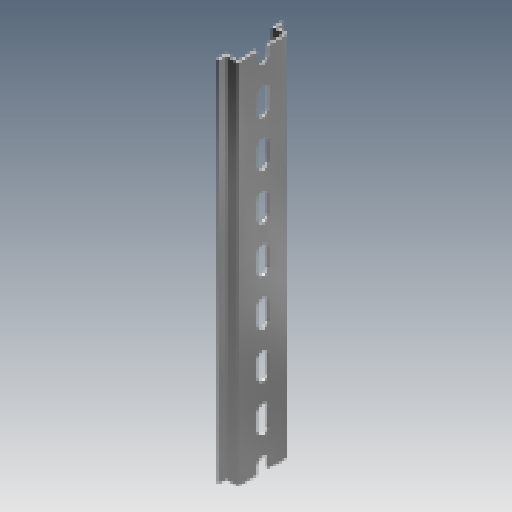
# Autodesk Inventor part: din_rail
Saved by Autodesk Inventor 2025.4 (Build 294407020, 407B)
## iProperties
Created: 2026-09-16
Part Number: din_rail
Material: Generic
Document SubType Name: Modeling
Designer: Aiden
Density: 1 g/cm^3
Appearance: Default
Author: Aiden
Autodesk Inventor part; units mm, degrees
ref_plane "YZ Plane" through (0, 0, 0) normal (1, 0, 0) x (0, 1, 0)
ref_plane "XZ Plane" through (0, 0, 0) normal (0, 1, 0) x (-1, 0, 0)
ref_plane "XY Plane" through (0, 0, 0) normal (0, 0, 1) x (1, 0, 0)
sketch "Sketch1" plane through (0, 0, 0) normal (0, 1, 0) x (-1, 0, 0)
  line L0 (0, 0) -> (0, -13.5)
  line L1 (0, -13.5) -> (6.5, -13.5)
  line L2 (6.5, -13.5) -> (6.5, -17.5)
  line L3 (1, 0) -> (1, -12.5)
  line L4 (1, -12.5) -> (7.5, -12.5)
  line L5 (7.5, -12.5) -> (7.5, -17.5)
  line L6 (7.5, -17.5) -> (6.5, -17.5)
  line L7 (1, 0) -> (0, 0) construction
  line L8 (0, 0) -> (0, 13.5)
  line L9 (0, 13.5) -> (6.5, 13.5)
  line L10 (6.5, 13.5) -> (6.5, 17.5)
  line L11 (1, 0) -> (1, 12.5)
  line L12 (1, 12.5) -> (7.5, 12.5)
  line L13 (7.5, 12.5) -> (7.5, 17.5)
  line L14 (7.5, 17.5) -> (6.5, 17.5)
  dimension "d0" = 13.5
  dimension "d1" = 1
  dimension "d2" = 7.5
  dimension "d3" = 17.5
  constraints: 30 end point, 6 symmetric about line, 3 horizontal, 2 vertical, 2 other
  measures "d0" distance of L0.start L0.end
  measures "d1" distance between parallel lines of L0 L3
  measures "d2" distance between parallel lines of L0 L5
  measures "d3" vertical distance of L2.end L0.start
extrude "Extrusion1" add sketch "Sketch1" along normal blind 200
sketch "Sketch2" plane through (-1, 0, -12.5) normal (-1, 0, 0) x (0, 0, 1)
  line L0 (0, 0) -> (25, 0) projected
  line L1 (25, 0) -> (25, 200) projected
  line L2 (0, 200) -> (25, 200) projected
  line L3 (0, 0) -> (0, 200) projected
  line L4 (25, 0) -> (25, 200) projected
  line L5 (12.5, 104.4) -> (12.5, 95.6) construction
  line L6 (30, 0) -> (30, 200) projected
  line L7 (9.4, 104.4) -> (9.4, 95.6)
  line L8 (15.6, 95.6) -> (15.6, 104.4)
  arc A0 (15.6, 104.4) -> (9.4, 104.4) centre (12.5, 104.4) ccw
  arc A1 (9.4, 95.6) -> (15.6, 95.6) centre (12.5, 95.6) ccw
  line L9 (12.5, 129.4) -> (12.5, 120.6) construction
  line L10 (9.4, 129.4) -> (9.4, 120.6)
  line L11 (15.6, 120.6) -> (15.6, 129.4)
  arc A2 (15.6, 129.4) -> (9.4, 129.4) centre (12.5, 129.4) ccw
  arc A3 (9.4, 120.6) -> (15.6, 120.6) centre (12.5, 120.6) ccw
  line L12 (12.5, 79.4) -> (12.5, 70.6) construction
  line L13 (9.4, 79.4) -> (9.4, 70.6)
  line L14 (15.6, 70.6) -> (15.6, 79.4)
  arc A4 (15.6, 79.4) -> (9.4, 79.4) centre (12.5, 79.4) ccw
  arc A5 (9.4, 70.6) -> (15.6, 70.6) centre (12.5, 70.6) ccw
  line L15 (12.5, 154.4) -> (12.5, 145.6) construction
  line L16 (9.4, 154.4) -> (9.4, 145.6)
  line L17 (15.6, 145.6) -> (15.6, 154.4)
  arc A6 (15.6, 154.4) -> (9.4, 154.4) centre (12.5, 154.4) ccw
  arc A7 (9.4, 145.6) -> (15.6, 145.6) centre (12.5, 145.6) ccw
  line L18 (12.5, 54.4) -> (12.5, 45.6) construction
  line L19 (9.4, 54.4) -> (9.4, 45.6)
  line L20 (15.6, 45.6) -> (15.6, 54.4)
  arc A8 (15.6, 54.4) -> (9.4, 54.4) centre (12.5, 54.4) ccw
  arc A9 (9.4, 45.6) -> (15.6, 45.6) centre (12.5, 45.6) ccw
  line L21 (12.5, 179.4) -> (12.5, 170.6) construction
  line L22 (9.4, 179.4) -> (9.4, 170.6)
  line L23 (15.6, 170.6) -> (15.6, 179.4)
  arc A10 (15.6, 179.4) -> (9.4, 179.4) centre (12.5, 179.4) ccw
  arc A11 (9.4, 170.6) -> (15.6, 170.6) centre (12.5, 170.6) ccw
  line L24 (12.5, 29.4) -> (12.5, 20.6) construction
  line L25 (9.4, 29.4) -> (9.4, 20.6)
  line L26 (15.6, 20.6) -> (15.6, 29.4)
  arc A12 (15.6, 29.4) -> (9.4, 29.4) centre (12.5, 29.4) ccw
  arc A13 (9.4, 20.6) -> (15.6, 20.6) centre (12.5, 20.6) ccw
  line L27 (12.5, 204.4) -> (12.5, 195.6) construction
  line L28 (9.4, 204.4) -> (9.4, 195.6)
  line L29 (15.6, 195.6) -> (15.6, 204.4)
  arc A14 (15.6, 204.4) -> (9.4, 204.4) centre (12.5, 204.4) ccw
  arc A15 (9.4, 195.6) -> (15.6, 195.6) centre (12.5, 195.6) ccw
  line L30 (12.5, 4.4) -> (12.5, -4.4) construction
  line L31 (9.4, 4.4) -> (9.4, -4.4)
  line L32 (15.6, -4.4) -> (15.6, 4.4)
  arc A16 (15.6, 4.4) -> (9.4, 4.4) centre (12.5, 4.4) ccw
  arc A17 (9.4, -4.4) -> (15.6, -4.4) centre (12.5, -4.4) ccw
  point P0 (12.5, 0)
  point P1 (12.5, 100)
  point P2 (12.5, 200)
  point P3 (25, 100)
  point P4 (12.5, 107.5)
  point P5 (12.5, 92.5)
  point P6 (12.5, 132.5)
  point P7 (12.5, 117.5)
  point P8 (12.5, 125)
  point P9 (12.5, 82.5)
  point P10 (12.5, 67.5)
  point P11 (12.5, 75)
  point P12 (12.5, 157.5)
  point P13 (12.5, 142.5)
  point P14 (12.5, 150)
  point P15 (12.5, 57.5)
  point P16 (12.5, 42.5)
  point P17 (12.5, 50)
  point P18 (12.5, 182.5)
  point P19 (12.5, 167.5)
  point P20 (12.5, 175)
  point P21 (12.5, 32.5)
  point P22 (12.5, 17.5)
  point P23 (12.5, 25)
  point P24 (12.5, 207.5)
  point P25 (12.5, 192.5)
  point P26 (12.5, 200)
  point P27 (12.5, 7.5)
  point P28 (12.5, -7.5)
  point P29 (12.5, 0)
  point P30 (9.4, 0)
  point P31 (15.6, 0)
  dimension "d6" = 6.2
  dimension "d7" = 15
  dimension "d10" = 25
  constraints: 72 end point, 38 point on circle, 18 centre point, 4 tangent, 3 midpoint, 2 parallel, 1 horizontal alignment, 1 vertical, 1 vertical alignment, 112 other
  measures "d6" distance between parallel lines of L7 L8
  measures "d7" distance of point (12.5, 107.5) point (12.5, 92.5)
  measures "d10" distance of L7.start L10.start
extrude "Extrusion2" cut sketch "Sketch2" against normal blind 15 contours L31 A16 L32 L0 | L28 A14 L29 L2 | L2 L29 A15 L28 | A0 L8 A1 L7 | A2 L11 A3 L10 | A4 L14 A5 L13 | A6 L17 A7 L16 | A8 L20 A9 L19 | A10 L23 A11 L22 | A12 L26 A13 L25
sketch "Sketch3" plane through (0, 200, 0) normal (0, 1, 0) x (1, 0, 0)
  line L0 (0, 3.1) -> (0, -3.1) projected
  line L1 (-1, -3.1) -> (-1, 3.1) projected
  line L2 (0, -3.1) -> (0, 3.1) projected
  line L3 (-1, -3.1) -> (0, -3.1) projected
  line L4 (-1, 3.1) -> (-1, -3.1) projected
  line L5 (-1, 3.1) -> (0, 3.1) projected
  line L6 (-1, -3.1) -> (0, -3.1) projected
  line L7 (-1, 3.1) -> (0, 3.1) projected
  line L8 (-1, 3.1) -> (0, 3.1) projected
  line L9 (0, 3.1) -> (0, -3.1) projected
  line L10 (-1, -3.1) -> (-1, 3.1) projected
  line L11 (0, 3.1) -> (0, -3.1) projected
  line L12 (-1, 3.1) -> (0, 3.1) projected
  line L13 (0, -3.1) -> (0, 3.1) projected
  line L14 (-1, -3.1) -> (0, -3.1) projected
  line L15 (-1, 3.1) -> (-1, -3.1) projected
  line L16 (-1, 3.1) -> (0, 3.1) projected
  line L17 (-1, -3.1) -> (-1, -12.5) projected
  line L18 (-1, -12.5) -> (-7.5, -12.5) projected
  line L19 (-7.5, -12.5) -> (-7.5, -17.5) projected
  line L20 (-7.5, -17.5) -> (-6.5, -17.5) projected
  line L21 (-6.5, -17.5) -> (-6.5, -13.5) projected
  line L22 (-6.5, -13.5) -> (0, -13.5) projected
  line L23 (0, -13.5) -> (0, -3.1) projected
  line L24 (0, 3.1) -> (0, 13.5) projected
  line L25 (0, 13.5) -> (-6.5, 13.5) projected
  line L26 (-6.5, 13.5) -> (-6.5, 17.5) projected
  line L27 (-6.5, 17.5) -> (-7.5, 17.5) projected
  line L28 (-7.5, 17.5) -> (-7.5, 12.5) projected
  line L29 (-7.5, 12.5) -> (-1, 12.5) projected
  line L30 (-1, 12.5) -> (-1, 3.1) projected
  line L31 (-1, -3.1) -> (0, -3.1) projected
  line L32 (-1, -3.1) -> (0, -3.1) projected
  line L33 (0, 3.1) -> (0, -3.1) projected
  line L34 (-1, 3.1) -> (0, 3.1) projected
  line L35 (-1, -3.1) -> (-1, 3.1) projected
  line L36 (-1, -3.1) -> (0, -3.1) projected
  line L37 (-1, 3.1) -> (0, 3.1) projected
  line L38 (-1, 3.1) -> (0, 3.1) projected
  line L39 (0, 3.1) -> (0, -3.1) projected
  line L40 (-1, 3.1) -> (0, 3.1) projected
  line L41 (-1, -3.1) -> (-1, 3.1) projected
  line L42 (-1, -3.1) -> (0, -3.1) projected
  line L43 (0, -3.1) -> (0, 3.1) projected
  line L44 (-1, -3.1) -> (0, -3.1) projected
  line L45 (-1, 3.1) -> (-1, -3.1) projected
  line L46 (-1, 3.1) -> (0, 3.1) projected
  line L47 (0, 3.1) -> (-1, 3.1) projected
  line L48 (-1, 12.5) -> (-1, 3.1) projected
  line L49 (-7.5, 12.5) -> (-1, 12.5) projected
  line L50 (-7.5, 17.5) -> (-7.5, 12.5) projected
  line L51 (-6.5, 17.5) -> (-7.5, 17.5) projected
  line L52 (-6.5, 13.5) -> (-6.5, 17.5) projected
  line L53 (0, 13.5) -> (-6.5, 13.5) projected
  line L54 (0, 3.1) -> (0, 13.5) projected
  line L55 (-1, -3.1) -> (0, -3.1) projected
  line L56 (-1, -3.1) -> (0, -3.1) projected
  line L57 (-1, -3.1) -> (0, -3.1) projected
  line L58 (0, -13.5) -> (0, -3.1) projected
  line L59 (-6.5, -13.5) -> (0, -13.5) projected
  line L60 (-6.5, -17.5) -> (-6.5, -13.5) projected
  line L61 (-7.5, -17.5) -> (-6.5, -17.5) projected
  line L62 (-7.5, -12.5) -> (-7.5, -17.5) projected
  line L63 (-1, -12.5) -> (-7.5, -12.5) projected
  line L64 (-1, -3.1) -> (-1, -12.5) projected
  line L65 (-1, -3.1) -> (0, -3.1) projected
  line L66 (-1, -3.1) -> (0, -3.1) projected
  line L67 (-1, -3.1) -> (0, -3.1) projected
  line L68 (-1, -3.1) -> (0, -3.1) projected
  line L69 (-1, 3.1) -> (0, 3.1) projected
  line L70 (-1, -3.1) -> (-1, 3.1) projected
  line L71 (0, 3.1) -> (0, -3.1) projected
  line L72 (0, 3.1) -> (0, -3.1) projected
  line L73 (-1, -3.1) -> (-1, 3.1) projected
  line L74 (-1, -3.1) -> (0, -3.1) projected
  line L75 (-1, 3.1) -> (0, 3.1) projected
  line L76 (-1, 3.1) -> (0, 3.1) projected
  line L77 (0, 3.1) -> (-1, 3.1) projected
  line L78 (0, 3.1) -> (-1, 3.1) projected
  line L79 (-1, -3.1) -> (0, -3.1) projected
  line L80 (-1, -3.1) -> (0, -3.1) projected
  line L81 (0, 3.1) -> (0, -3.1) projected
  line L82 (-1, -3.1) -> (-1, -12.5) projected
  line L83 (-1, -3.1) -> (-1, -12.5) projected
  line L84 (-1, -3.1) -> (-1, 3.1) projected
  line L85 (-1, 12.5) -> (-1, 3.1) projected
  line L86 (-1, 12.5) -> (-1, 3.1) projected
  line L87 (-1, 3.1) -> (-1, -3.1) projected
  line L88 (-1, -3.1) -> (-1, 3.1) projected
  line L89 (-1, 3.1) -> (-1, -3.1) projected
  line L90 (-1, -3.1) -> (-1, 3.1) projected
  line L91 (-1, 3.1) -> (-1, -3.1) projected
  line L92 (-1, -3.1) -> (-1, 3.1) projected
  line L93 (-1, 3.1) -> (-1, -3.1) projected
  line L94 (-1, -3.1) -> (-1, 3.1) projected
  line L95 (-1, 3.1) -> (-1, -3.1) projected
  line L96 (-1, -3.1) -> (-1, 3.1) projected
  line L97 (-1, 3.1) -> (-1, -3.1) projected
  line L98 (-1, -3.1) -> (-1, 3.1) projected
  line L99 (-1, 3.1) -> (-1, -3.1) projected
  line L100 (-1, -3.1) -> (-1, 3.1) projected
  line L101 (-1, 3.1) -> (-1, -3.1) projected
  line L102 (0, -3.1) -> (0, 3.1) projected
  line L103 (0, 3.1) -> (0, -3.1) projected
  line L104 (0, -3.1) -> (0, 3.1) projected
  line L105 (0, 3.1) -> (0, -3.1) projected
  line L106 (0, -3.1) -> (0, 3.1) projected
  line L107 (0, 3.1) -> (0, -3.1) projected
  line L108 (0, -3.1) -> (0, 3.1) projected
  line L109 (0, 3.1) -> (0, -3.1) projected
  line L110 (0, -3.1) -> (0, 3.1) projected
  line L111 (0, 3.1) -> (0, -3.1) projected
  line L112 (0, -3.1) -> (0, 3.1) projected
  line L113 (0, 3.1) -> (0, -3.1) projected
  line L114 (0, -3.1) -> (0, 3.1) projected
  line L115 (0, 3.1) -> (0, -3.1) projected
  line L116 (0, -3.1) -> (0, 3.1) projected
  line L117 (0, 3.1) -> (0, 13.5) projected
  line L118 (0, 3.1) -> (0, 13.5) projected
  line L119 (0, 3.1) -> (0, -3.1) projected
  line L120 (0, -13.5) -> (0, -3.1) projected
  line L121 (0, -13.5) -> (0, -3.1) projected
  line L122 (-1, 12.5) -> (-1, 3.1) projected
  line L123 (0, 3.1) -> (0, 13.5) projected
  line L124 (-7.5, 12.5) -> (-1, 12.5) projected
  line L125 (-7.5, 12.5) -> (-1, 12.5) projected
  line L126 (0, 13.5) -> (-6.5, 13.5) projected
  line L127 (0, 13.5) -> (-6.5, 13.5) projected
  line L128 (0, 13.5) -> (-6.5, 13.5) projected
  line L129 (-6.5, 13.5) -> (-6.5, 17.5) projected
  line L130 (-6.5, 13.5) -> (-6.5, 17.5) projected
  line L131 (-6.5, 13.5) -> (-6.5, 17.5) projected
  line L132 (-6.5, 17.5) -> (-7.5, 17.5) projected
  line L133 (-6.5, 17.5) -> (-7.5, 17.5) projected
  line L134 (-7.5, 17.5) -> (-7.5, 12.5) projected
  line L135 (-7.5, 17.5) -> (-7.5, 12.5) projected
  line L136 (-7.5, 17.5) -> (-7.5, 12.5) projected
  line L137 (-1, -3.1) -> (-1, 3.1) projected
  line L138 (-6.5, 17.5) -> (-7.5, 17.5) projected
  line L139 (-6.5, -13.5) -> (0, -13.5) projected
  line L140 (-7.5, 12.5) -> (-1, 12.5) projected
  line L141 (-1, -12.5) -> (-7.5, -12.5) projected
  line L142 (-1, -3.1) -> (0, -3.1) projected
  line L143 (-1, -3.1) -> (-1, -12.5) projected
  line L144 (0, -13.5) -> (0, -3.1) projected
  line L145 (-1, -12.5) -> (-7.5, -12.5) projected
  line L146 (-1, -12.5) -> (-7.5, -12.5) projected
  line L147 (-6.5, -13.5) -> (0, -13.5) projected
  line L148 (-6.5, -13.5) -> (0, -13.5) projected
  line L149 (-7.5, -12.5) -> (-7.5, -17.5) projected
  line L150 (-7.5, -12.5) -> (-7.5, -17.5) projected
  line L151 (-7.5, -12.5) -> (-7.5, -17.5) projected
  line L152 (-6.5, -17.5) -> (-6.5, -13.5) projected
  line L153 (-6.5, -17.5) -> (-6.5, -13.5) projected
  line L154 (-6.5, -17.5) -> (-6.5, -13.5) projected
  line L155 (-7.5, -17.5) -> (-6.5, -17.5) projected
  line L156 (-7.5, -17.5) -> (-6.5, -17.5) projected
  line L157 (-7.5, -17.5) -> (-6.5, -17.5) projected
  line L158 (-1, -3.1) -> (-1, 3.1) projected
  line L159 (-1, -3.1) -> (0, -3.1) projected
  line L160 (0, 3.1) -> (0, -3.1) projected
  line L161 (-1, 3.1) -> (0, 3.1) projected
  line L162 (-1, -3.1) -> (-1, 3.1) projected
  line L163 (-1, -3.1) -> (0, -3.1) projected
  line L164 (-1, 3.1) -> (0, 3.1) projected
  line L165 (-1, 3.1) -> (0, 3.1) projected
  line L166 (-1, 3.1) -> (0, 3.1) projected
  line L167 (0, -3.1) -> (0, 3.1) projected
  line L168 (-1, -3.1) -> (0, -3.1) projected
  line L169 (-1, 3.1) -> (-1, -3.1) projected
  line L170 (-1, 3.1) -> (0, 3.1) projected
  line L171 (-1, -3.1) -> (-1, 3.1) projected
  line L172 (0, 3.1) -> (0, -3.1) projected
  line L173 (-1, 3.1) -> (0, 3.1) projected
  line L174 (0, 3.1) -> (0, -3.1) projected
  line L175 (-1, 3.1) -> (0, 3.1) projected
  line L176 (-1, -3.1) -> (-1, 3.1) projected
  line L177 (-1, -3.1) -> (0, -3.1) projected
  line L178 (-1, -3.1) -> (-1, 3.1) projected
  line L179 (0, 3.1) -> (0, -3.1) projected
  line L180 (-1, -3.1) -> (0, -3.1) projected
  line L181 (-1, 3.1) -> (0, 3.1) projected
  line L182 (0, 3.1) -> (0, -3.1) projected
  line L183 (-1, 3.1) -> (0, 3.1) projected
  line L184 (-1, 3.1) -> (0, 3.1) projected
  line L185 (-1, -3.1) -> (-1, 3.1) projected
  line L186 (-1, -3.1) -> (0, -3.1) projected
  line L187 (-1, -3.1) -> (0, -3.1) projected
  line L188 (-1, 3.1) -> (0, 3.1) projected
  line L189 (-1, 3.1) -> (0, 3.1) projected
  line L190 (0, -3.1) -> (0, 3.1) projected
  line L191 (-1, -3.1) -> (0, -3.1) projected
  line L192 (-1, 3.1) -> (-1, -3.1) projected
  line L193 (-1, 3.1) -> (0, 3.1) projected
  line L194 (-1, 3.1) -> (0, 3.1) projected
  line L195 (-1, -3.1) -> (-1, 3.1) projected
  line L196 (0, 3.1) -> (0, -3.1) projected
  line L197 (-1, -3.1) -> (-1, 3.1) projected
  line L198 (0, 3.1) -> (0, -3.1) projected
  line L199 (-1, -3.1) -> (0, -3.1) projected
  line L200 (-1, 3.1) -> (0, 3.1) projected
  line L201 (-1, 3.1) -> (0, 3.1) projected
  line L202 (-1, 3.1) -> (0, 3.1) projected
  line L203 (-1, -3.1) -> (-1, 3.1) projected
  line L204 (0, 3.1) -> (0, -3.1) projected
  line L205 (-1, 3.1) -> (0, 3.1) projected
  line L206 (-1, -3.1) -> (0, -3.1) projected
  line L207 (-1, 3.1) -> (0, 3.1) projected
  line L208 (-1, -3.1) -> (0, -3.1) projected
  line L209 (-1, -3.1) -> (-1, 3.1) projected
  line L210 (0, 3.1) -> (0, -3.1) projected
  line L211 (0, 3.1) -> (0, -3.1) projected
  line L212 (-1, 3.1) -> (0, 3.1) projected
  line L213 (-1, -3.1) -> (-1, 3.1) projected
  line L214 (-1, -3.1) -> (0, -3.1) projected
  line L215 (-1, -3.1) -> (0, -3.1) projected
  line L216 (0, 3.1) -> (0, -3.1) projected
  line L217 (-1, -3.1) -> (-1, 3.1) projected
  line L218 (0, 3.1) -> (0, -3.1) projected
  line L219 (0, -3.1) -> (-1, -3.1) projected
  line L220 (-1, -3.1) -> (0, -3.1) projected
  line L221 (-1, -3.1) -> (-1, 3.1) projected
  line L222 (-1, 3.1) -> (0, 3.1) projected
  line L223 (-1, 3.1) -> (0, 3.1) projected
  line L224 (0, -3.1) -> (-1, -3.1) projected
  line L225 (-1, -3.1) -> (-1, -12.5) projected
  line L226 (-1, -12.5) -> (-7.5, -12.5) projected
  line L227 (-7.5, -12.5) -> (-7.5, -17.5) projected
  line L228 (-7.5, -17.5) -> (-6.5, -17.5) projected
  line L229 (-6.5, -17.5) -> (-6.5, -13.5) projected
  line L230 (-6.5, -13.5) -> (0, -13.5) projected
  line L231 (0, -13.5) -> (0, -3.1) projected
  line L232 (-1, 3.1) -> (0, 3.1) projected
  line L233 (0, 3.1) -> (0, 13.5) projected
  line L234 (0, 13.5) -> (-6.5, 13.5) projected
  line L235 (-6.5, 13.5) -> (-6.5, 17.5) projected
  line L236 (-6.5, 17.5) -> (-7.5, 17.5) projected
  line L237 (-7.5, 17.5) -> (-7.5, 12.5) projected
  line L238 (-7.5, 12.5) -> (-1, 12.5) projected
  line L239 (-1, 12.5) -> (-1, 3.1) projected
  line L240 (0, -3.1) -> (0, 3.1) projected
  line L241 (-1, -3.1) -> (0, -3.1) projected
  line L242 (-1, 3.1) -> (-1, -3.1) projected
  line L243 (-1, 3.1) -> (0, 3.1) projected
  line L244 (0, 3.1) -> (0, -3.1) projected
  line L245 (-1, 3.1) -> (0, 3.1) projected
  line L246 (-1, -3.1) -> (-1, 3.1) projected
  line L247 (-1, -3.1) -> (0, -3.1) projected
  line L248 (-1, -3.1) -> (0, -3.1) projected
  line L249 (-1, -3.1) -> (0, -3.1) projected
  line L250 (0, 3.1) -> (0, -3.1) projected
  line L251 (-1, 3.1) -> (0, 3.1) projected
  line L252 (-1, -3.1) -> (-1, 3.1) projected
  line L253 (-1, -3.1) -> (0, -3.1) projected
  line L254 (-1, -3.1) -> (0, -3.1) projected
  line L255 (-1, -3.1) -> (0, -3.1) projected
  line L256 (-1, 3.1) -> (0, 3.1) projected
  line L257 (-1, 3.1) -> (0, 3.1) projected
  line L258 (0, -3.1) -> (0, 3.1) projected
  line L259 (-1, -3.1) -> (0, -3.1) projected
  line L260 (-1, 3.1) -> (-1, -3.1) projected
  line L261 (-1, 3.1) -> (0, 3.1) projected
  line L262 (0, 3.1) -> (0, -3.1) projected
  line L263 (-1, 3.1) -> (0, 3.1) projected
  line L264 (-1, -3.1) -> (-1, 3.1) projected
  line L265 (-1, -3.1) -> (0, -3.1) projected
  line L266 (-1, -3.1) -> (0, -3.1) projected
  line L267 (-1, -3.1) -> (0, -3.1) projected
  line L268 (-1, 3.1) -> (0, 3.1) projected
  line L269 (-1, 3.1) -> (0, 3.1) projected
  line L270 (0, -3.1) -> (0, 3.1) projected
  line L271 (-1, -3.1) -> (0, -3.1) projected
  line L272 (-1, 3.1) -> (-1, -3.1) projected
  line L273 (-1, 3.1) -> (0, 3.1) projected
  line L274 (0, 3.1) -> (0, -3.1) projected
  line L275 (-1, 3.1) -> (0, 3.1) projected
  line L276 (-1, -3.1) -> (-1, 3.1) projected
  line L277 (-1, -3.1) -> (0, -3.1) projected
  line L278 (0, -3.1) -> (-1, -3.1) projected
  line L279 (-1, -3.1) -> (0, -3.1) projected
  line L280 (-1, 3.1) -> (0, 3.1) projected
  line L281 (-1, 3.1) -> (0, 3.1) projected
  line L282 (-1, 3.1) -> (0, 3.1) projected
  line L283 (-1, 3.1) -> (0, 3.1) projected
  line L284 (-1, -3.1) -> (0, -3.1) projected
  line L285 (-1, -3.1) -> (0, -3.1) projected
  line L286 (-1, -3.1) -> (0, -3.1) projected
  line L287 (-1, -3.1) -> (0, -3.1) projected
  point P0 (0, 0)
  constraints: 56 vertical, 28 perpendicular, 24 horizontal, 37 other
equation "\"d15\" = d7"
body "Solid1"
